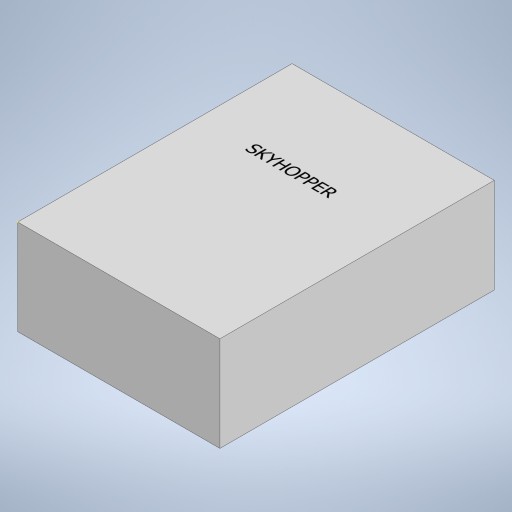
# Autodesk Inventor part: skyhopper
Saved by Autodesk Inventor 2023 (Build 270158000, 158)
## iProperties
Created: 2022-08-11
Part Number: skyhopper
Material: Generic
Document SubType Name: Modeling
Designer: Eli
Density: 1 g/cm^3
Appearance: Default
Author: Eli
Autodesk Inventor part; units mm, degrees
ref_plane "YZ Plane" through (0, 0, 0) normal (1, 0, 0) x (0, 1, 0)
ref_plane "XZ Plane" through (0, 0, 0) normal (0, 1, 0) x (-1, 0, 0)
ref_plane "XY Plane" through (0, 0, 0) normal (0, 0, 1) x (1, 0, 0)
sketch "Sketch1" plane through (0, 0, 0) normal (0, 1, 0) x (-1, 0, 0)
  line L0 (0, 0) -> (-54.102, 0)
  line L1 (-54.102, 0) -> (-54.102, -73.406)
  line L2 (-54.102, -73.406) -> (0, -73.406)
  line L3 (0, -73.406) -> (0, 0)
  dimension "d0" = 73.406
  dimension "d1" = 54.102
  constraints: 8 end point, 2 parallel, 1 horizontal, 1 perpendicular
  measures "d0" distance of L2.end L0.start
  measures "d1" distance of L1.end L2.end
extrude "Extrusion1" add sketch "Sketch1" along normal blind 25.4
sketch "Sketch2" plane through (0, 25.4, 0) normal (0, 1, 0) x (1, 0, 0)
  line L0 (13.483, 50.1527) -> (44.1688, 50.1527) construction
  line L1 (44.1688, 50.1527) -> (44.1688, 23.7266) construction
  line L2 (44.1688, 23.7266) -> (13.483, 23.7266) construction
  line L3 (13.483, 23.7266) -> (13.483, 50.1527) construction
  point P0 (0, 0)
  constraints: 2 other
body "Solid1"
